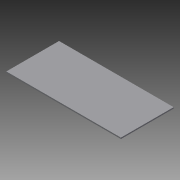
# Autodesk Inventor part: large wall
Saved by Autodesk Inventor 2015 (Build 190159000, 159)
## iProperties
Created: 2015-01-31
Part Number: large wall
Material: Generic
Document SubType Name: Modeling
Designer: Joseph
Density: 1 g/cm^3
Appearance: Default
Author: Joseph
Autodesk Inventor part; units mm, degrees
ref_plane "YZ Plane" through (0, 0, 0) normal (1, 0, 0) x (0, 1, 0)
ref_plane "XZ Plane" through (0, 0, 0) normal (0, 1, 0) x (-1, 0, 0)
ref_plane "XY Plane" through (0, 0, 0) normal (0, 0, 1) x (1, 0, 0)
sketch "Sketch1" plane through (0, 0, 0) normal (0, 0, 1) x (1, 0, 0)
  line L0 (0, -18.0326) -> (20, -18.0326) projected
  line L1 (20, 0) -> (20, -18.0326) projected
  line L2 (-580, 258.0326) -> (-500, 258.0326) projected
  line L3 (-580, 240) -> (-580, 258.0326) projected
  line L4 (20, -18.0326) -> (-580, -18.0326)
  line L5 (-580, -18.0326) -> (-580, 258.0326)
  line L6 (-580, 258.0326) -> (20, 258.0326)
  line L7 (20, 258.0326) -> (20, -18.0326)
  point P0 (0, 0)
  constraints: 8 end point, 2 parallel, 1 horizontal, 1 perpendicular
extrude "Extrusion1" add sketch "Sketch1" along normal blind 6.35
body "Solid1"
